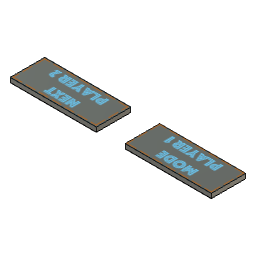
button_nameplates (Autodesk Fusion 360 design; units mm, degrees)
Autodesk Fusion 360 part; units mm, degrees
sketch "plate1" plane through (0, 0, 0) normal (0, 0, 1) x (1, 0, 0)
  line L0 (0, 0) -> (-75, 0)
  line L1 (-75, 0) -> (-75, 30)
  line L2 (-75, 30) -> (0, 30)
  line L3 (0, 30) -> (0, 0)
  dimension "d1" = 75
  dimension "d2" = 30
  constraint horizontal L0
  constraint vertical L1
  constraint horizontal L2
  constraint vertical L3
  constraint coincident L0.start L3.end
  measures "d1" distance of L0.start L0.end
  measures "d2" distance of L0.start L2.end
extrude "Extrude1" add sketch "plate1" along normal blind 4 makes body 1
sketch "plate2" plane through (0, 0, 0) normal (0, 0, 1) x (1, 0, 0)
  line L0 (-65.0278, -0.0817) -> (-140.0278, -0.0817)
  line L1 (-140.0278, -0.0817) -> (-140.0278, 29.9183)
  line L2 (-140.0278, 29.9183) -> (-65.0278, 29.9183)
  line L3 (-65.0278, 29.9183) -> (-65.0278, -0.0817)
  dimension "d6" = 75
  dimension "d7" = 30
  constraint horizontal L0
  constraint vertical L1
  constraint horizontal L2
  constraint vertical L3
  measures "d6" distance of L0.start L0.end
  measures "d7" distance of L0.start L2.end
extrude "Extrude2" add sketch "plate2" along normal blind 4 separate body makes body 2
move_body "Move1" bodies 2 to x (1, 0, 0) y (0, 1, 0) z (0, 0, 1) at (-35, 0, 0)
sketch "Sketch10" plane through (0, 0, 4) normal (0, 0, 1) x (-1, 0, 0)
  line L0 (0, -30) -> (75, -30)
  line L1 (75, -30) -> (75, 0)
  line L2 (75, 0) -> (0, 0)
  line L3 (0, 0) -> (0, -30)
  line L4 (1.0793, -29.3064) -> (74.2846, -29.3064) construction
  line L5 (74.2846, -29.3064) -> (74.2846, -0.9988) construction
  line L6 (74.2846, -0.9988) -> (1.0793, -0.9988) construction
  line L7 (1.0793, -0.9988) -> (1.0793, -29.3064) construction
  dimension "d12" = 8
sketch "Sketch11" plane through (0, 0, 4) normal (0, 0, 1) x (-1, 0, 0)
  line L0 (100.0278, -29.9183) -> (175.0278, -29.9183)
  line L1 (175.0278, -29.9183) -> (175.0278, 0.0817)
  line L2 (175.0278, 0.0817) -> (100.0278, 0.0817)
  line L3 (100.0278, 0.0817) -> (100.0278, -29.9183)
  line L4 (101.6596, -28.7579) -> (173.8208, -28.7579) construction
  line L5 (173.8208, -28.7579) -> (173.8208, -1.2624) construction
  line L6 (173.8208, -1.2624) -> (101.6596, -1.2624) construction
  line L7 (101.6596, -1.2624) -> (101.6596, -28.7579) construction
  dimension "d13" = 8
